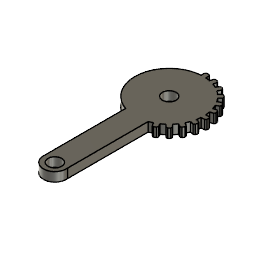
Gear Linkage (Autodesk Fusion 360 design; units mm, degrees)
part number: 2026-03-10-21-41-45-371
Autodesk Fusion 360 part; units mm, degrees
sketch "Sketch1" plane through (0, 0, 0) normal (0, 0, 1) x (1, 0, 0)
  circle A0 centre (-33.9346, 12.5591) radius 3
  line L0 (-38.896, 13.1793) -> (-38.896, 48.4001)
  line L1 (-28.9732, 13.1793) -> (-28.9732, 48.3974)
  line L2 (-34.9607, 77.5191) -> (-34.9607, 79.0591)
  line L3 (-32.9007, 77.5191) -> (-32.8964, 79.0591)
  arc A1 (-38.896, 13.1793) -> (-28.9732, 13.1793) centre (-33.9346, 12.5591) ccw
  line L4 (-34.4286, 79.5291) -> (-33.4286, 79.5291)
  line L5 (-34.9607, 79.0591) -> (-34.4286, 79.5291)
  line L6 (-32.8964, 79.0591) -> (-33.4286, 79.5291)
  line L7 (-25.5564, 50.1097) -> (-24.7864, 48.7761)
  line L8 (-24.7864, 48.7761) -> (-25.0123, 48.103)
  line L9 (-25.0123, 48.103) -> (-25.8783, 47.603)
  line L10 (-26.5742, 47.7439) -> (-25.8783, 47.603)
  line L11 (-27.3405, 49.0797) -> (-26.5742, 47.7439)
  line L12 (-22.6209, 52.7012) -> (-21.5319, 51.6123)
  line L13 (-21.5319, 51.6123) -> (-21.5759, 50.9036)
  line L14 (-21.5759, 50.9036) -> (-22.283, 50.1965)
  line L15 (-22.9916, 50.1526) -> (-22.283, 50.1965)
  line L16 (-24.0775, 51.2446) -> (-22.9916, 50.1526)
  line L17 (-20.456, 55.9642) -> (-19.1223, 55.1942)
  line L18 (-19.1223, 55.1942) -> (-18.9814, 54.4983)
  line L19 (-18.9814, 54.4983) -> (-19.4814, 53.6323)
  line L20 (-20.1545, 53.4064) -> (-19.4814, 53.6323)
  line L21 (-21.486, 54.1802) -> (-20.1545, 53.4064)
  line L22 (-19.2095, 59.6762) -> (-17.7219, 59.2777)
  line L23 (-17.7219, 59.2777) -> (-17.4057, 58.642)
  line L24 (-17.4057, 58.642) -> (-17.6645, 57.6761)
  line L25 (-18.2562, 57.2837) -> (-17.6645, 57.6761)
  line L26 (-19.7426, 57.6864) -> (-18.2562, 57.2837)
  line L27 (-18.9661, 63.5845) -> (-17.4261, 63.5845)
  line L28 (-17.4261, 63.5845) -> (-16.9561, 63.0523)
  line L29 (-16.9561, 63.0523) -> (-16.9561, 62.0523)
  line L30 (-17.4261, 61.5201) -> (-16.9561, 62.0523)
  line L31 (-18.9661, 61.5245) -> (-17.4261, 61.5201)
  line L32 (-19.7426, 67.4225) -> (-18.2551, 67.8211)
  line L33 (-18.2551, 67.8211) -> (-17.6634, 67.4287)
  line L34 (-17.6634, 67.4287) -> (-17.4046, 66.4628)
  line L35 (-17.7208, 65.8271) -> (-17.4046, 66.4628)
  line L36 (-19.2095, 65.4327) -> (-17.7208, 65.8271)
  line L37 (-21.486, 70.9288) -> (-20.1523, 71.6988)
  line L38 (-20.1523, 71.6988) -> (-19.4792, 71.4729)
  line L39 (-19.4792, 71.4729) -> (-18.9792, 70.6069)
  line L40 (-19.1202, 69.911) -> (-18.9792, 70.6069)
  line L41 (-20.456, 69.1448) -> (-19.1202, 69.911)
  line L42 (-24.0775, 73.8644) -> (-22.9886, 74.9533)
  line L43 (-22.9886, 74.9533) -> (-22.2799, 74.9093)
  line L44 (-22.2799, 74.9093) -> (-21.5728, 74.2022)
  line L45 (-21.5288, 73.4936) -> (-21.5728, 74.2022)
  line L46 (-22.6209, 72.4077) -> (-21.5288, 73.4936)
  line L47 (-27.3405, 76.0292) -> (-26.5705, 77.3629)
  line L48 (-26.5705, 77.3629) -> (-25.8746, 77.5038)
  line L49 (-25.8746, 77.5038) -> (-25.0086, 77.0038)
  line L50 (-24.7827, 76.3307) -> (-25.0086, 77.0038)
  line L51 (-25.5564, 74.9992) -> (-24.7827, 76.3307)
  line L52 (-31.0525, 77.2757) -> (-30.6539, 78.7633)
  line L53 (-30.6539, 78.7633) -> (-30.0183, 79.0795)
  line L54 (-30.0183, 79.0795) -> (-29.0523, 78.8207)
  line L55 (-28.66, 78.229) -> (-29.0523, 78.8207)
  line L56 (-29.0627, 76.7426) -> (-28.66, 78.229)
  arc A2 (-31.0525, 77.2757) -> (-32.9007, 77.5191) centre (-33.9307, 62.5545) ccw
  arc A3 (-27.3405, 76.0292) -> (-29.0627, 76.7426) centre (-33.9307, 62.5545) ccw
  arc A4 (-24.0775, 73.8644) -> (-25.5564, 74.9992) centre (-33.9307, 62.5545) ccw
  arc A5 (-21.486, 70.9288) -> (-22.6209, 72.4077) centre (-33.9307, 62.5545) ccw
  arc A6 (-19.7426, 67.4225) -> (-20.456, 69.1448) centre (-33.9307, 62.5545) ccw
  arc A7 (-18.9661, 63.5845) -> (-19.2095, 65.4327) centre (-33.9307, 62.5545) ccw
  arc A8 (-19.2095, 59.6762) -> (-18.9661, 61.5245) centre (-33.9307, 62.5545) ccw
  arc A9 (-20.456, 55.9642) -> (-19.7426, 57.6864) centre (-33.9307, 62.5545) ccw
  arc A10 (-25.5564, 50.1097) -> (-24.0775, 51.2446) centre (-33.9307, 62.5545) ccw
  arc A11 (-22.6209, 52.7012) -> (-21.486, 54.1802) centre (-33.9307, 62.5545) ccw
  arc A12 (-34.9607, 77.5191) -> (-38.896, 48.4001) centre (-33.9307, 62.5545) ccw
  arc A13 (-28.9732, 48.3974) -> (-27.3405, 49.0797) centre (-33.9307, 62.5545) ccw
  dimension "d5" = 6
  dimension "d6" = 10
  dimension "d10" = 2.06
  dimension "d11" = 1.54
  dimension "d12" = 1.54
  dimension "d23" = 1
  dimension "d24" = 0.47
  dimension "d25" = 0.47
  dimension "d26" = 0.71
  dimension "d27" = 0.71
  dimension "d28" = 30
  dimension "d30" = 360
  dimension "d31" = 66.97
  constraint concentric A0 A1
  constraint vertical L0
  constraint parallel L0 L1
  constraint vertical L2
  constraint horizontal L4
  constraint concentric A2 A12
  constraint concentric A2 A3
  constraint concentric A3 A4
  constraint concentric A4 A5
  constraint concentric A5 A6
  constraint concentric A6 A7
  constraint concentric A7 A8
  constraint concentric A8 A9
  constraint concentric A9 A11
  constraint concentric A10 A11
  constraint concentric A12 A13
  measures "d5" diameter of A0
  measures "d6" diameter of A1
  measures "d10" distance of L2.start L3.start
  measures "d11" distance of L2.start L2.end
  measures "d12" distance of L3.start L3.end
  measures "d23" distance of L4.start L4.end
  measures "d24" distance of L2.end L4
  measures "d25" distance of L3.end L4
  measures "d26" distance of L3.end L4.end
  measures "d27" distance of L2.end L4.start
  measures "d28" diameter of A10
  measures "d31" distance of A0.centre L4
extrude "Extrude1" add sketch "Sketch1" along normal blind 4
sketch "Sketch2" plane through (0, 0, 0) normal (0, 0, 1) x (1, 0, 0)
sketch "Sketch3" plane through (0, 0, 0) normal (1, 0, 0) x (0, 1, 0)
sketch "Sketch4" plane through (0, 0, 0) normal (0, 0, 1) x (1, 0, 0)
sketch "Sketch5" plane through (0, 0, 4) normal (0, 0, 1) x (-1, 0, 0)
  circle A0 centre (33.9346, -12.5591) radius 3
  arc A1 (38.896, -13.1793) -> (28.9732, -13.1793) centre (33.9346, -12.5591) ccw
  line L0 (28.9732, -13.1793) -> (28.9732, -48.3974)
  arc A2 (28.9732, -48.3974) -> (27.3405, -49.0797) centre (33.9307, -62.5545) ccw
  line L1 (27.3405, -49.0797) -> (26.5742, -47.7439)
  line L2 (26.5742, -47.7439) -> (25.8783, -47.603)
  line L3 (25.8783, -47.603) -> (25.0123, -48.103)
  line L4 (25.0123, -48.103) -> (24.7864, -48.7761)
  line L5 (24.7864, -48.7761) -> (25.5564, -50.1097)
  arc A3 (25.5564, -50.1097) -> (24.0775, -51.2446) centre (33.9307, -62.5545) ccw
  line L6 (24.0775, -51.2446) -> (22.9916, -50.1526)
  line L7 (22.9916, -50.1526) -> (22.283, -50.1965)
  line L8 (22.283, -50.1965) -> (21.5759, -50.9036)
  line L9 (21.5759, -50.9036) -> (21.5319, -51.6123)
  line L10 (21.5319, -51.6123) -> (22.6209, -52.7012)
  arc A4 (22.6209, -52.7012) -> (21.486, -54.1802) centre (33.9307, -62.5545) ccw
  line L11 (21.486, -54.1802) -> (20.1545, -53.4064)
  line L12 (20.1545, -53.4064) -> (19.4814, -53.6323)
  line L13 (19.4814, -53.6323) -> (18.9814, -54.4983)
  line L14 (18.9814, -54.4983) -> (19.1223, -55.1942)
  line L15 (19.1223, -55.1942) -> (20.456, -55.9642)
  arc A5 (20.456, -55.9642) -> (19.7426, -57.6864) centre (33.9307, -62.5545) ccw
  line L16 (19.7426, -57.6864) -> (18.2562, -57.2837)
  line L17 (18.2562, -57.2837) -> (17.6645, -57.6761)
  line L18 (17.6645, -57.6761) -> (17.4057, -58.642)
  line L19 (17.4057, -58.642) -> (17.7219, -59.2777)
  line L20 (17.7219, -59.2777) -> (19.2095, -59.6762)
  arc A6 (19.2095, -59.6762) -> (18.9661, -61.5245) centre (33.9307, -62.5545) ccw
  line L21 (18.9661, -61.5245) -> (17.4261, -61.5201)
  line L22 (17.4261, -61.5201) -> (16.9561, -62.0523)
  line L23 (16.9561, -62.0523) -> (16.9561, -63.0523)
  line L24 (16.9561, -63.0523) -> (17.4261, -63.5845)
  line L25 (17.4261, -63.5845) -> (18.9661, -63.5845)
  arc A7 (18.9661, -63.5845) -> (19.2095, -65.4327) centre (33.9307, -62.5545) ccw
  line L26 (19.2095, -65.4327) -> (17.7208, -65.8271)
  line L27 (17.7208, -65.8271) -> (17.4046, -66.4628)
  line L28 (17.4046, -66.4628) -> (17.6634, -67.4287)
  line L29 (17.6634, -67.4287) -> (18.2551, -67.8211)
  line L30 (18.2551, -67.8211) -> (19.7426, -67.4225)
  arc A8 (19.7426, -67.4225) -> (20.456, -69.1448) centre (33.9307, -62.5545) ccw
  line L31 (20.456, -69.1448) -> (19.1202, -69.911)
  line L32 (19.1202, -69.911) -> (18.9792, -70.6069)
  line L33 (18.9792, -70.6069) -> (19.4792, -71.4729)
  line L34 (19.4792, -71.4729) -> (20.1523, -71.6988)
  line L35 (20.1523, -71.6988) -> (21.486, -70.9288)
  arc A9 (21.486, -70.9288) -> (22.6209, -72.4077) centre (33.9307, -62.5545) ccw
  line L36 (22.6209, -72.4077) -> (21.5288, -73.4936)
  line L37 (21.5288, -73.4936) -> (21.5728, -74.2022)
  line L38 (21.5728, -74.2022) -> (22.2799, -74.9093)
  line L39 (22.2799, -74.9093) -> (22.9886, -74.9533)
  line L40 (22.9886, -74.9533) -> (24.0775, -73.8644)
  arc A10 (24.0775, -73.8644) -> (25.5564, -74.9992) centre (33.9307, -62.5545) ccw
  line L41 (25.5564, -74.9992) -> (24.7827, -76.3307)
  line L42 (24.7827, -76.3307) -> (25.0086, -77.0038)
  line L43 (25.0086, -77.0038) -> (25.8746, -77.5038)
  line L44 (25.8746, -77.5038) -> (26.5705, -77.3629)
  line L45 (26.5705, -77.3629) -> (27.3405, -76.0292)
  arc A11 (27.3405, -76.0292) -> (29.0627, -76.7426) centre (33.9307, -62.5545) ccw
  line L46 (29.0627, -76.7426) -> (28.66, -78.229)
  line L47 (28.66, -78.229) -> (29.0523, -78.8207)
  line L48 (29.0523, -78.8207) -> (30.0183, -79.0795)
  line L49 (30.0183, -79.0795) -> (30.6539, -78.7633)
  line L50 (30.6539, -78.7633) -> (31.0525, -77.2757)
  arc A12 (31.0525, -77.2757) -> (32.9007, -77.5191) centre (33.9307, -62.5545) ccw
  line L51 (32.9007, -77.5191) -> (32.8964, -79.0591)
  line L52 (32.8964, -79.0591) -> (33.4286, -79.5291)
  line L53 (33.4286, -79.5291) -> (34.4286, -79.5291)
  line L54 (34.4286, -79.5291) -> (34.9607, -79.0591)
  line L55 (34.9607, -79.0591) -> (34.9607, -77.5191)
  arc A13 (34.9607, -77.5191) -> (38.896, -48.4001) centre (33.9307, -62.5545) ccw
  line L56 (38.896, -48.4001) -> (38.896, -13.1793)
  circle A14 centre (33.9307, -62.5545) radius 3
  dimension "d32" = 6
  constraint concentric A2 A14
  measures "d32" diameter of A14
extrude "Extrude2" cut sketch "Sketch5" against normal blind 20 contours A14
